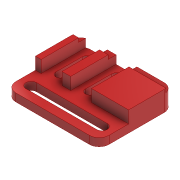
# Autodesk Inventor part: Limit switch mount top nut well
Saved by Autodesk Inventor 2020 (Build 240168000, 168)
## iProperties
Created: 2019-11-30
Part Number: Limit switch mount top nut well
Material: Generic
Document SubType Name: Modeling
Designer: ball
Density: 1 g/cm^3
Appearance: Default
Author: ball
Autodesk Inventor part; units mm, degrees
ref_plane "YZ Plane" through (0, 0, 0) normal (1, 0, 0) x (0, 1, 0)
sketch "Sketch1" plane through (0, 0, 0) normal (0, 1, 0) x (-1, 0, 0)
  line L0 (0, 0) -> (30.0482, 0)
  line L1 (30.0482, 0) -> (30.0482, -24.13)
  line L2 (30.0482, -24.13) -> (0, -24.13)
  line L3 (0, -24.13) -> (0, 0)
  line L4 (15.3416, -12.2936) -> (15.3416, -20.8026) construction
  line L5 (13.9319, -12.2936) -> (13.9319, -20.8026)
  line L6 (16.7513, -20.8026) -> (16.7513, -12.2936)
  arc A0 (16.7513, -12.2936) -> (13.9319, -12.2936) centre (15.3416, -12.2936) ccw
  arc A1 (13.9319, -20.8026) -> (16.7513, -20.8026) centre (15.3416, -20.8026) ccw
  line L7 (24.8666, -12.2936) -> (24.8666, -20.8026) construction
  line L8 (23.4569, -12.2936) -> (23.4569, -20.8026)
  line L9 (26.2763, -20.8026) -> (26.2763, -12.2936)
  arc A2 (26.2763, -12.2936) -> (23.4569, -12.2936) centre (24.8666, -12.2936) ccw
  arc A3 (23.4569, -20.8026) -> (26.2763, -20.8026) centre (24.8666, -20.8026) ccw
  line L10 (26.4414, -4.4958) -> (3.6068, -4.4958) construction
  line L11 (26.4414, -2.7958) -> (3.6068, -2.7958)
  line L12 (3.6068, -6.1958) -> (26.4414, -6.1958)
  arc A4 (26.4414, -6.1958) -> (26.4414, -2.7958) centre (26.4414, -4.4958) ccw
  arc A5 (3.6068, -2.7958) -> (3.6068, -6.1958) centre (3.6068, -4.4958) ccw
  point P0 (15.3416, -16.5481)
  point P1 (24.8666, -16.5481)
  point P2 (15.0241, -4.4958)
  dimension "d0" = 30.0482
  dimension "d1" = 24.13
  dimension "d5" = 12.2936
  dimension "d6" = 2.8194
  dimension "d8" = 3.3274
  dimension "d11" = 9.525
  dimension "d16" = 3.4
  dimension "d17" = 4.4958
  dimension "d18" = 3.6068
  dimension "d19" = 3.6068
  dimension "d43" = 5.1816
  constraints: 32 end point, 12 point on circle, 8 tangent, 6 centre point, 5 parallel, 2 horizontal, 2 midpoint, 1 perpendicular, 1 vertical, 12 other
  measures "d0" distance of L1.end L2.end
  measures "d1" distance of L0.end L1.end
  measures "d5" distance from line of L0 L4.start
  measures "d6" diameter of A1
  measures "d8" distance from line of L2 L4.end
  measures "d11" distance of L5.start L8.start
  measures "d16" diameter of A5
  measures "d17" distance from line of L0 L10.end
  measures "d18" distance from line of L1 L10.start
  measures "d19" distance from line of L3 L10.end
  measures "d43" distance from line of L1 point (24.867, -16.548)
extrude "Shape" add sketch "Sketch1" along normal blind 2.54
sketch "Sketch2" plane through (0, 2.54, 0) normal (0, 1, 0) x (1, 0, 0)
  line L0 (0, 24.13) -> (-30.0482, 24.13) projected
  line L1 (0, 0) -> (0, 24.13) projected
  line L2 (-30.0482, 24.13) -> (0, 24.13)
  line L3 (0, 24.13) -> (0, 9.5)
  line L4 (0, 9.5) -> (-30.0482, 9.5)
  line L5 (-30.0482, 9.5) -> (-30.0482, 24.13)
  line L6 (-30.0482, 0) -> (0, 0) projected
  line L7 (-11.9634, 9.5) -> (-11.9634, 24.13)
  line L8 (-11.9634, 24.13) -> (-18.6944, 24.13)
  line L9 (-18.6944, 24.13) -> (-18.6944, 9.5)
  arc A0 (-16.7513, 12.2936) -> (-13.9319, 12.2936) centre (-15.3416, 12.2936) ccw projected
  line L10 (-18.1778, 2.3562) -> (-11.9634, 24.13) construction
  line L11 (-12.9982, 4.0205) -> (-18.6944, 24.13) construction
  line L12 (-18.6944, 9.5) -> (-1.5875, 9.5)
  line L13 (-28.2194, 24.13) -> (-28.2194, 9.5)
  line L14 (-21.4884, 9.5) -> (-21.4884, 24.13)
  line L15 (-28.2194, 9.5) -> (-11.1125, 9.5)
  line L16 (-21.4884, 24.13) -> (-28.2194, 24.13)
  point P0 (-11.9634, 24.13)
  point P1 (-21.4884, 9.5)
  point P2 (-18.6944, 9.5)
  point P3 (-28.2194, 24.13)
  dimension "d22" = 9.5
  dimension "d23" = 6.731
  dimension "d27" = 9.525
  dimension "d44" = 1.8288
  constraints: 28 end point, 5 point on line, 3 collinear, 3 parallel, 2 horizontal, 2 perpendicular, 9 other
  measures "d22" distance between parallel lines of L6 L4
  measures "d23" distance between parallel lines of L7 L9
  measures "d27" distance of L8.end L13.start
  measures "d44" distance between parallel lines of L5 L13
extrude "Extrusion2" add sketch "Sketch2" along normal blind 3.937 contours L1 L4 L7 L0 | L9 L4 L14 L0 | L13 L4 L5 L0
ref_plane "Work Plane1" through (-15.3416, 0, -12.2936) normal (1, 0, 0) x (0, 0, -1)
ref_plane "Work Plane2" through (-24.8666, 0, -12.2936) normal (1, 0, 0) x (0, 0, -1)
sketch "Sketch3" plane through (0, 0, 0) normal (1, 0, 0) x (0, 0, -1)
  line L0 (24.13, 6.477) -> (9.5, 6.477) projected
  line L1 (24.13, 6.477) -> (21.59, 6.477)
  line L2 (21.59, 6.477) -> (21.59, 5.207)
  line L3 (21.59, 5.207) -> (24.13, 5.207)
  line L4 (24.13, 5.207) -> (24.13, 6.477)
  point P0 (0, 0)
  dimension "d35" = 2.54
  dimension "d36" = 1.27
  constraints: 8 end point, 2 parallel, 1 horizontal, 1 perpendicular
  measures "d35" distance of L3.end L2.end
  measures "d36" distance of L2.end L1.end
extrude "Extrusion3" cut sketch "Sketch3" against normal through all
fillet "Fillet2" radius 3.175 4 edges at (0, 1.27, 0) (0, 2.6035, -24.13) (-30.0482, 2.6035, -24.13) (-30.0482, 1.27, 0)
equation "\"d19\" = d18"
equation "\"d27\" = d11"
body "Solid1"
